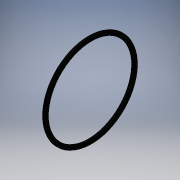
# Autodesk Inventor part: O Ring 72x3,5x65
Saved by Autodesk Inventor 2017.3 (Build 213256000, 256)
## iProperties
Created: 2017-11-10
Part Number: O Ring 72x3,5x65
Material: Eisen, grau
Document SubType Name: Modeling
Designer: Christoph Soppa
Density: 7.15 g/cm^3
Appearance: Eloxiert - schwarz
Author: Christoph Soppa
Autodesk Inventor part; units mm, degrees
ref_plane "YZ Plane" through (0, 0, 0) normal (1, 0, 0) x (0, 1, 0)
ref_plane "XZ Plane" through (0, 0, 0) normal (0, 1, 0) x (-1, 0, 0)
ref_plane "XY Plane" through (0, 0, 0) normal (0, 0, 1) x (1, 0, 0)
sketch "Skizze1" plane through (0, 0, 0) normal (0, 0, 1) x (1, 0, 0)
  circle A0 centre (0, 34.25) radius 1.75
  line L0 (-21.28, 0) -> (17.2096, 0) projected
  line L1 (0, -7.2) -> (0, 43.2) projected
  line L2 (-15.7815, 0) -> (11.7111, 0)
  point P0 (0, 0)
  dimension "d1" = 3.5
  dimension "d2" = 34.25
  dimension "d3" = 0
  constraints: 2 end point, 2 point on line, 1 centre point
  measures "d1" diameter of A0
  measures "d2" distance from line of A0.centre L0
  measures "d3" distance from line of L1 A0.centre
revolve "Umdrehung1" add sketch "Skizze1" angle 360 about axis through (-15.7815, 0, 0) along (1, 0, 0)
